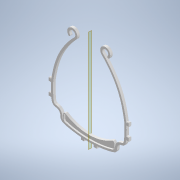
# Autodesk Inventor part: headband
Saved by Autodesk Inventor 2020 (Build 240168000, 168)
## iProperties
Created: 2020-03-27
Part Number: headband
Material: Generic
Document SubType Name: Modeling
Designer: Clevo
Density: 1 g/cm^3
Appearance: Default
Author: Clevo
Autodesk Inventor part; units mm, degrees
ref_plane "YZ Plane" through (0, 0, 0) normal (1, 0, 0) x (0, 1, 0)
ref_plane "XZ Plane" through (0, 0, 0) normal (0, 1, 0) x (-1, 0, 0)
ref_plane "XY Plane" through (0, 0, 0) normal (0, 0, 1) x (1, 0, 0)
sketch "Sketch2" plane through (0, 0, 0) normal (0, 0, 1) x (1, 0, 0)
  line L0 (0, -29.928708) -> (16.20738, -29.928708) construction
  line L1 (16.20738, -29.928708) -> (31.17577, -27.4689) construction
  line L2 (31.17577, -27.4689) -> (40.898711, -25.355218) construction
  line L3 (40.898711, -25.355218) -> (45.266988, -24.157464) construction
  spline S0 degree 4 poles (0, -29.928708) (16.20738, -29.928708) (31.17577, -27.4689) (40.898711, -25.355218) (45.266988, -24.157464) knots 1 1 1 1 1 2 2 2 2 2
  line L4 (45.266988, -24.157464) -> (52.576045, -21.872268) construction
  line L5 (52.576045, -21.872268) -> (53.375446, -20.906724) construction
  line L6 (53.375446, -20.906724) -> (57.17737, -17.047635) construction
  line L7 (57.17737, -17.047635) -> (55.67911, -11.751982) construction
  line L8 (55.67911, -11.751982) -> (57.995671, -5.271128) construction
  line L9 (57.995671, -5.271128) -> (63.355591, -2.697056) construction
  line L10 (63.355591, -2.697056) -> (68.318745, -2.857693) construction
  line L11 (68.318745, -2.857693) -> (72.734904, 0.406423) construction
  line L12 (72.734904, 0.406423) -> (73.895575, 4.930064) construction
  line L13 (73.895575, 4.930064) -> (74.222943, 9.632269) construction
  spline S1 degree 4 poles (45.266988, -24.157464) (52.576045, -21.872268) (53.375446, -20.906724) (57.17737, -17.047635) (55.67911, -11.751982) (57.995671, -5.271128) (63.355591, -2.697056) (68.318745, -2.857693) (72.734904, 0.406423) (73.895575, 4.930064) (74.222943, 9.632269) knots 1 1 1 1 1 2 3 4 5 6 7 8 8 8 8 8
  line L14 (74.222943, 9.632269) -> (75.79954, 32.277938) construction
  line L15 (75.79954, 32.277938) -> (74.222943, 43.703978) construction
  line L16 (74.222943, 43.703978) -> (70.505758, 64.71395) construction
  line L17 (70.505758, 64.71395) -> (62.725192, 86.726478) construction
  line L18 (62.725192, 86.726478) -> (55.67911, 101.819369) construction
  line L19 (55.67911, 101.819369) -> (40.252249, 124.473776) construction
  line L20 (40.252249, 124.473776) -> (28.5, 135.895585) construction
  spline S2 degree 4 poles (74.222943, 9.632269) (75.79954, 32.277938) (74.222943, 43.703978) (70.505758, 64.71395) (62.725192, 86.726478) (55.67911, 101.819369) (40.252249, 124.473776) (28.5, 135.895585) knots 1 1 1 1 1 2 3 4 5 5 5 5 5
  arc A0 (36.311578, 135.315802) -> (28.5, 135.895585) centre (32.742229, 140.138637) ccw
  point P0 (0, 0)
  dimension "d4" = 16.20738
  dimension "d5" = 31.17577
  dimension "d6" = 40.89871
  dimension "d7" = 52.57605
  dimension "d8" = 53.37545
  dimension "d9" = 55.67911
  dimension "d10" = 57.17737
  dimension "d11" = 57.99567
  dimension "d12" = 63.35559
  dimension "d13" = 68.31875
  dimension "d14" = 72.7349
  dimension "d15" = 73.89557
  dimension "d16" = 75.79954
  dimension "d17" = 74.22294
  dimension "d18" = 70.50576
  dimension "d19" = 62.72519
  dimension "d20" = 55.67911
  dimension "d21" = 40.25225
  dimension "d22" = 32.74223
  dimension "d23" = 29.92871
  dimension "d24" = 29.92871
  dimension "d25" = 27.4689
  dimension "d26" = 25.35522
  dimension "d27" = 21.87227
  dimension "d28" = 20.90672
  dimension "d29" = 17.04764
  dimension "d30" = 11.75198
  dimension "d31" = 5.27113
  dimension "d32" = 2.69706
  dimension "d33" = 2.85769
  dimension "d34" = 0.40642
  dimension "d35" = 4.93006
  dimension "d36" = 32.27794
  dimension "d37" = 43.70398
  dimension "d38" = 64.71395
  dimension "d39" = 86.72648
  dimension "d40" = 101.81937
  dimension "d41" = 124.47378
  dimension "d42" = 140.13864
  dimension "d43" = 6
  dimension "d44" = 28.5
  dimension "d45" = 135.89558
  dimension "d46" = 9.63227
  dimension "d47" = 74.22294
  dimension "d48" = 45.26699
  dimension "d49" = 24.15746
  constraints: 2 point on circle, 1 centre point, 1 horizontal, 1 vertical alignment, 9 other
  measures "d4" horizontal distance of point (0, 0) L0.end
  measures "d5" horizontal distance of point (0, 0) L1.end
  measures "d6" horizontal distance of point (0, 0) L2.end
  measures "d7" horizontal distance of point (0, 0) L4.end
  measures "d8" horizontal distance of point (0, 0) L5.end
  measures "d9" horizontal distance of point (0, 0) L7.end
  measures "d10" horizontal distance of point (0, 0) L6.end
  measures "d11" horizontal distance of point (0, 0) L8.end
  measures "d12" horizontal distance of point (0, 0) L9.end
  measures "d13" horizontal distance of point (0, 0) L10.end
  measures "d14" horizontal distance of point (0, 0) L11.end
  measures "d15" horizontal distance of point (0, 0) L12.end
  measures "d16" horizontal distance of point (0, 0) L14.end
  measures "d17" horizontal distance of point (0, 0) L15.end
  measures "d18" horizontal distance of point (0, 0) L16.end
  measures "d19" horizontal distance of point (0, 0) L17.end
  measures "d20" horizontal distance of point (0, 0) L18.end
  measures "d21" horizontal distance of point (0, 0) L19.end
  measures "d22" horizontal distance of point (0, 0) A0.centre
  measures "d23" distance of point (0, 0) L0.start
  measures "d24" vertical distance of point (0, 0) L0.end
  measures "d25" vertical distance of point (0, 0) L1.end
  measures "d26" vertical distance of point (0, 0) L2.end
  measures "d27" vertical distance of point (0, 0) L4.end
  measures "d28" vertical distance of point (0, 0) L5.end
  measures "d29" vertical distance of point (0, 0) L6.end
  measures "d30" vertical distance of point (0, 0) L7.end
  measures "d31" vertical distance of point (0, 0) L8.end
  measures "d32" vertical distance of point (0, 0) L9.end
  measures "d33" vertical distance of point (0, 0) L10.end
  measures "d34" vertical distance of point (0, 0) L11.end
  measures "d35" vertical distance of point (0, 0) L12.end
  measures "d36" vertical distance of point (0, 0) L14.end
  measures "d37" vertical distance of point (0, 0) L15.end
  measures "d38" vertical distance of point (0, 0) L16.end
  measures "d39" vertical distance of point (0, 0) L17.end
  measures "d40" vertical distance of point (0, 0) L18.end
  measures "d41" vertical distance of point (0, 0) L19.end
  measures "d42" vertical distance of point (0, 0) A0.centre
  measures "d43" radius of A0
  measures "d44" horizontal distance of point (0, 0) L20.end
  measures "d45" vertical distance of point (0, 0) L20.end
  measures "d46" vertical distance of point (0, 0) L13.end
  measures "d47" horizontal distance of point (0, 0) L13.end
  measures "d48" horizontal distance of L3.end point (0, 0)
  measures "d49" vertical distance of point (0, 0) L3.end
ref_plane "Work Plane1" through (0, 0, 0) normal (-1, 0, 0) x (0, -1, 0)
sketch "Sketch3" plane through (0, 0, 0) normal (-1, 0, 0) x (0, -1, 0)
  line L0 (29.928708, 0) -> (25.928708, 0)
  line L1 (25.928708, 0) -> (25.928708, 5)
  line L2 (25.928708, 5) -> (29.928708, 5)
  line L3 (29.928708, 5) -> (29.928708, 0)
  point P0 (0, 0)
  dimension "d50" = 4
  dimension "d51" = 5
  constraints: 8 end point, 2 parallel, 1 horizontal, 1 perpendicular
  measures "d50" distance of L1.end L2.end
  measures "d51" distance of L2.end L0.start
sweep "Sweep1" add profiles "Sketch3" path "Sketch2"
fillet "Fillet1" radius 2 2 edges at (38.6911, 132.1006, 2.5) (36.3116, 135.3158, 2.5)
sketch "Sketch5" plane through (0, 0, 0) normal (0, 0, 1) x (1, 0, 0)
  circle A0 centre (0, 70) radius 87.5
  line L0 (50.290517, -1.603868) -> (51.413253, -15.752043)
  line L1 (51.413253, -15.752043) -> (51.088771, -18.16992) construction
  line L2 (51.088771, -18.16992) -> (48.963649, -19.232481) construction
  spline S0 degree 2 poles (51.413253, -15.752043) (51.088771, -18.16992) (48.963649, -19.232481) knots 1 1 1 2 2 2
  line L3 (48.963649, -19.232481) -> (39.334201, -23.139162)
  line L4 (39.334201, -23.139162) -> (0, -27.576164)
  line L5 (0, -27.576164) -> (0, -17.5)
  line L6 (0, -25.928708) -> (0, -29.928708)
  point P0 (0, 0)
  dimension "d56" = 175
  dimension "d57" = 70
  dimension "d58" = 50.29052
  dimension "d59" = 1.60387
  dimension "d60" = 51.41325
  dimension "d61" = 15.75204
  dimension "d62" = 51.08877
  dimension "d63" = 18.16992
  dimension "d64" = 48.96365
  dimension "d65" = 19.23248
  dimension "d66" = 39.3342
  dimension "d67" = 23.13916
  dimension "d68" = 27.57616
  constraints: 8 end point, 2 point on circle, 2 vertical alignment, 1 centre point, 1 collinear, 3 other
  measures "d56" diameter of A0
  measures "d57" distance of point (0, 0) A0.centre
  measures "d58" horizontal distance of point (0, 0) L0.start
  measures "d59" vertical distance of point (0, 0) L0.start
  measures "d60" horizontal distance of point (0, 0) L0.end
  measures "d61" vertical distance of point (0, 0) L0.end
  measures "d62" horizontal distance of point (0, 0) L1.end
  measures "d63" vertical distance of point (0, 0) L1.end
  measures "d64" horizontal distance of point (0, 0) L2.end
  measures "d65" vertical distance of point (0, 0) L2.end
  measures "d66" horizontal distance of point (0, 0) L3.end
  measures "d67" vertical distance of point (0, 0) L3.end
  measures "d68" distance of point (0, 0) L4.end
extrude "Extrusion2" add sketch "Sketch5" along normal up to surface (5 mm away) contours A0 L0 S0 L3 L4 L5
fillet "Fillet2" radius 3 1 edges at (50.2905, -1.6039, 2.5)
sketch "Sketch8" plane through (0, -29.928708, 5) normal (0, 0, 1) x (1, 0, 0)
  line L0 (16.570216, 6.091793) -> (8.770216, 6.091793)
  line L1 (8.770216, 6.091793) -> (8.770216, -3.608207)
  line L2 (8.770216, -3.608207) -> (16.570216, -3.608207)
  line L3 (16.570216, -3.608207) -> (16.570216, 6.091793)
  line L4 (79.341805, 39.278248) -> (71.640677, 39.278248)
  line L5 (71.640677, 39.278248) -> (71.640677, 47.296482)
  line L6 (71.640677, 47.296482) -> (79.341805, 47.296482)
  line L7 (79.341805, 47.296482) -> (79.341805, 39.278248)
  line L8 (79.341805, 64.700451) -> (76.59381, 64.700451)
  line L9 (76.59381, 64.700451) -> (76.59381, 72.609193)
  line L10 (76.59381, 72.609193) -> (79.341805, 72.609193)
  line L11 (79.341805, 72.609193) -> (79.341805, 64.700451)
  line L12 (76.59381, 64.700451) -> (71.640677, 64.700451)
  line L13 (71.640677, 64.700451) -> (71.640677, 71.65668)
  line L14 (71.640677, 71.65668) -> (76.59381, 71.65668)
  line L15 (76.59381, 71.65668) -> (76.59381, 64.700451)
  point P0 (0, 29.928708)
  point P1 (76.59381, 71.65668)
  dimension "d84" = 7.8
  dimension "d85" = 8.77022
  dimension "d86" = 23.83691
  dimension "d87" = 9.7
  dimension "d88" = 7.70113
  dimension "d89" = 8.01823
  dimension "d90" = 7.90874
  dimension "d91" = 6.95623
  dimension "d92" = 4.95313
  dimension "d93" = 2.748
  dimension "d94" = 71.64068
  dimension "d95" = 9.34954
  dimension "d96" = 34.77174
  constraints: 32 end point, 8 parallel, 4 horizontal, 4 perpendicular, 2 point on line
  measures "d84" distance of L1.end L2.end
  measures "d85" distance from line of point (0, 29.929) L1
  measures "d86" distance from line of point (0, 29.929) L0
  measures "d87" distance of L0.end L1.end
  measures "d88" distance of L4.start L4.end
  measures "d89" distance of L6.end L4.start
  measures "d90" distance of L10.end L8.start
  measures "d91" distance of L12.end L13.end
  measures "d92" distance of L13.end L14.end
  measures "d93" distance of L9.end L10.end
  measures "d94" distance from line of L5 point (0, 29.929)
  measures "d95" distance from line of L4 point (0, 29.929)
  measures "d96" distance from line of point (0, 29.929) L12
extrude "Extrusion4" add sketch "Sketch8" against normal up to surface (5 mm away) separate body
sketch "Sketch10" plane through (79.341805, 34.771744, 5) normal (1, 0, 0) x (0, 0, -1)
  line L0 (5, 0) -> (5, 7.908741)
  line L1 (0, 7.908741) -> (5, 7.908741)
  line L2 (0, 0) -> (0, 7.908741)
  line L3 (0, 0) -> (5, 0)
  circle A0 centre (2.5, 4.208741) radius 3.7
  circle A1 centre (2.5, 3.7) radius 3.7
  line L4 (0, 0) -> (5, 0)
  line L5 (0, 7.908741) -> (5, 7.908741)
  line L6 (5, 7.908741) -> (5, 6.956228)
  line L7 (0, 0) -> (5, 0)
  line L8 (5, 7.908741) -> (0, 7.908741)
  line L9 (0, 7.908741) -> (0, 0)
  line L10 (0, 0) -> (5, 0)
  line L11 (5, 0) -> (5, 7.908741)
  point P0 (5, -34.771744)
  point P1 (2.5, 0)
  point P2 (2.5, 0)
  point P3 (0, 0.972364)
  point P4 (5, 0.972364)
  point P5 (0, 6.936377)
  point P6 (2.5, 7.908741)
  point P7 (5, 6.936377)
  dimension "d102" = 7.4
  dimension "d103" = 7.4
  constraints: 8 end point, 2 centre point, 2 parallel, 2 tangent, 2 vertical alignment, 1 horizontal, 1 midpoint, 1 perpendicular
  measures "d102" diameter of A0
  measures "d103" diameter of A1
fillet "Fillet4" radius 2.5 2 edges at (74.1172, 41.728, 0) (74.1172, 41.728, 5)
extrude "Extrusion5" cut sketch "Sketch10" against normal through all contours L0 A0 L1 | A0 L2 L1 | L0 L3 A1 | A1 L3 L2 bodies 2
sketch "Sketch11" plane through (79.341805, 9.349541, 5) normal (1, 0, 0) x (0, 0, -1)
  line L0 (5, 0) -> (5, 8.018234)
  line L1 (0, 8.018234) -> (5, 8.018234)
  line L2 (0, 0) -> (0, 8.018234)
  line L3 (0, 0) -> (5, 0)
  circle A0 centre (2.5, 4.318234) radius 3.7
  circle A1 centre (2.5, 3.7) radius 3.7
  line L4 (0, 0) -> (5, 0)
  line L5 (0, 8.018234) -> (5, 8.018234)
  line L6 (5, 8.018234) -> (0, 8.018234)
  line L7 (0, 8.018234) -> (0, 0)
  line L8 (0, 0) -> (5, 0)
  line L9 (5, 0) -> (5, 8.018234)
  point P0 (5, -9.349541)
  point P1 (2.5, 0)
  point P2 (2.5, 0)
  point P3 (0, 0.972364)
  point P4 (5, 0.972364)
  point P5 (0, 7.04587)
  point P6 (2.5, 8.018234)
  point P7 (5, 7.04587)
  dimension "d107" = 7.4
  dimension "d108" = 7.4
  constraints: 8 end point, 2 centre point, 2 parallel, 2 tangent, 2 vertical alignment, 1 horizontal, 1 midpoint, 1 perpendicular
  measures "d107" diameter of A0
  measures "d108" diameter of A1
extrude "Extrusion6" cut sketch "Sketch11" against normal through all contours L3 A1 L0 | L3 L2 A1 | A0 L1 L0 | L2 L1 A0 bodies 2
sketch "Sketch12" plane through (8.770216, -33.536914, 5) normal (0, -1, 0) x (1, 0, 0)
  line L0 (0, -5) -> (7.8, -5) projected
  line L1 (7.8, 0) -> (7.8, -5) projected
  line L2 (0, 0) -> (7.8, 0) projected
  line L3 (0, 0) -> (0, -5) projected
  line L4 (7.8, -5) -> (0, -5)
  line L5 (0, -5) -> (0, 0)
  line L6 (0, 0) -> (7.8, 0)
  line L7 (7.8, 0) -> (7.8, -5)
  circle A0 centre (4.1, -2.5) radius 3.7
  circle A1 centre (3.7, -2.5) radius 3.7
  point P0 (-8.770216, -5)
  point P1 (7.8, -2.5)
  point P2 (0, -2.5)
  point P3 (0.972364, 0)
  point P4 (0.972364, -5)
  point P5 (6.827636, 0)
  point P6 (7.8, -2.5)
  point P7 (6.827636, -5)
  dimension "d111" = 7.4
  dimension "d112" = 7.4
  constraints: 8 end point, 2 centre point, 2 horizontal alignment, 2 parallel, 2 tangent, 1 horizontal, 1 midpoint, 1 perpendicular
  measures "d111" diameter of A0
  measures "d112" diameter of A1
extrude "Extrusion7" cut sketch "Sketch12" against normal through all contours L3 A1 L0 | L3 L2 A1 | A0 L1 L0 | A0 L2 L1 bodies 2
combine bodies "Combine1" operation type add bodies to combine 1 2
sketch "Sketch13" plane through (79.341805, 10.321904, 5) normal (0, 0, 1) x (1, 0, 0)
  line L0 (-28.649244, -16.992144) -> (-27.928552, -26.073948)
  arc A0 (-28.649244, -16.992144) -> (-33.221123, -14.680042) centre (-31.639842, -17.229464) ccw
  arc A1 (-79.341805, -27.821904) -> (-33.221123, -14.680042) centre (-79.341805, 59.678096) ccw
  line L1 (-29.437443, -26.021335) -> (-30.144543, -17.110804)
  arc A2 (-30.144543, -17.110804) -> (-32.430483, -15.954753) centre (-31.639842, -17.229464) ccw
  arc A3 (-79.341805, -29.321904) -> (-32.430483, -15.954753) centre (-79.341805, 59.678096) ccw
  line L2 (-29.437443, -26.021335) -> (-30.962901, -29.321904)
  line L3 (-30.962901, -29.321904) -> (-40.478894, -32.311091) construction
  line L4 (-40.478894, -32.311091) -> (-56.994423, -35.606198) construction
  line L5 (-56.994423, -35.606198) -> (-69.939948, -36.354031) construction
  line L6 (-69.939948, -36.354031) -> (-77.31457, -36.354031) construction
  line L7 (-79.341805, -27.821904) -> (-79.341805, -40.250612)
  line L8 (-77.31457, -36.354031) -> (-79.341805, -36.354031) construction
  spline S0 degree 4 poles (-30.962901, -29.321904) (-40.478894, -32.311091) (-56.994423, -35.606198) (-69.939948, -36.354031) (-77.31457, -36.354031) (-79.341805, -36.354031) knots 1 1 1 1 1 2 3 3 3 3 3
  point P0 (-79.341805, -10.321904)
  dimension "d115" = 1.5
  dimension "d116" = 48.3789
  dimension "d117" = 19
  dimension "d118" = 38.86291
  dimension "d119" = 22.34738
  dimension "d120" = 9.40186
  dimension "d121" = 2.02724
  dimension "d122" = 26.03213
  dimension "d123" = 26.03213
  dimension "d124" = 25.28429
  dimension "d125" = 21.98919
  dimension "d126" = 49.90436
  constraints: 4 end point, 4 point on circle, 2 centre point, 1 horizontal, 1 point on line, 6 other
  measures "d115" distance between parallel lines of L0 L1
  measures "d116" horizontal distance of point (-79.342, -10.322) L2.end
  measures "d117" vertical distance of point (-79.342, -10.322) L2.end
  measures "d118" horizontal distance of point (-79.342, -10.322) L3.end
  measures "d119" horizontal distance of point (-79.342, -10.322) L4.end
  measures "d120" horizontal distance of point (-79.342, -10.322) L5.end
  measures "d121" horizontal distance of point (-79.342, -10.322) L6.end
  measures "d122" distance of point (-79.342, -10.322) L8.end
  measures "d123" vertical distance of point (-79.342, -10.322) L5.end
  measures "d124" vertical distance of point (-79.342, -10.322) L4.end
  measures "d125" vertical distance of point (-79.342, -10.322) L3.end
  measures "d126" horizontal distance of point (-79.342, -10.322) L1.start
extrude "Extrusion8" cut sketch "Sketch13" against normal blind 3 bodies 1
mirror "Mirror1" about plane through (0, -27.928708, 2.5) normal (-1, 0, 0) bodies 1
equation "\"d103\" = d102"
equation "\"d108\" = d107"
equation "\"d112\" = d111"
body "Solid2"
